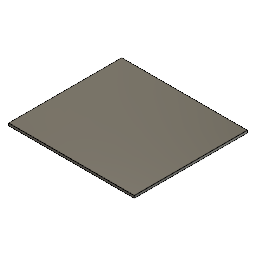
back v1 (Autodesk Fusion 360 design; units mm, degrees)
Autodesk Fusion 360 part; units mm, degrees
box "BoxPrimitive1" add length 90 width 100 height 2 placed x (0, 0, 1) y (1, 0, 0) z (0, 1, 0) at (0, 0, 0)
